Eufy Camera Corner Mount (Autodesk Fusion 360 design; units mm, degrees)
Autodesk Fusion 360 part; units mm, degrees
sketch "Sketch1" plane through (0, 0, 0) normal (0, 0, 1) x (1, 0, 0)
  line L0 (0, 0) -> (0, -37.5335) construction
  line L1 (31.3, -31.3) -> (31.3, 13.7)
  line L2 (31.3, -31.3) -> (2, -2)
  line L3 (-31.3, -31.3) -> (-31.3, 13.7)
  line L4 (-31.3, -31.3) -> (-2, -2)
  line L5 (31.3, 13.7) -> (-31.3, 13.7)
  arc A0 (2, -2) -> (-2, -2) centre (0, -2) ccw
  dimension "d1" = 62.6
  dimension "d2" = 45
  dimension "d4" = 90
  dimension "d5" = 2
  constraint coincident L0.start origin
  constraint vertical L0
  constraint vertical L1
  constraint symmetric L0 L1.start L3.start
  constraint symmetric L0 L1.end L3.end
  constraint coincident L0.start A0
  constraint midpoint L0.start A0
  constraint equal L2 L4
  constraint vertical L0.start A0.centre
  constraint horizontal L2.end A0.centre
  measures "d1" distance of L1.end L3.end
  measures "d2" distance of L1.start L1.end
  measures "d4" angle of L2 L4
  measures "d5" radius of A0
extrude "Extrude1" add sketch "Sketch1" along normal blind 56
sketch "Sketch2" plane through (0, 0, 0) normal (0.707107, -0.707107, 0) x (0.707107, 0.707107, 0)
  line L0 (-44.2649, 0) -> (-2.8284, 0)
  line L1 (-2.8284, 0) -> (-2.8284, 56)
  line L2 (-2.8284, 56) -> (-44.2649, 56)
  line L3 (-44.2649, 56) -> (-44.2649, 0)
  circle A0 centre (-25.8284, 41) radius 2
  circle A1 centre (-25.8284, 15) radius 2
  circle A2 centre (-25.8284, 15) radius 6.5
  circle A3 centre (-25.8284, 41) radius 6.5
  dimension "d8" = 15
  dimension "d10" = 4
  dimension "d11" = 15
  dimension "d12" = 23
  dimension "d15" = 13
  constraint equal A0 A1
  constraint vertical A0.centre A1.centre
  constraint concentric A1 A2
  constraint concentric A0 A3
  constraint equal A2 A3
  measures "d8" distance of L2 A0.centre
  measures "d10" diameter of A1
  measures "d11" distance of L0 A1.centre
  measures "d12" distance of L1 A0.centre
  measures "d15" diameter of A2
extrude "Extrude2" cut sketch "Sketch2" against normal blind 61.002 contours A0 | A1
extrude "Extrude3" cut sketch "Sketch2" along normal blind 17 from surface at -30 contours A2 | A3
sketch "Sketch3" plane through (0, 13.7, 0) normal (0, 1, 0) x (-1, 0, 0)
  line L0 (-31.3, 0) -> (31.3, 0)
  line L1 (31.3, 0) -> (31.3, 56)
  line L2 (31.3, 56) -> (-31.3, 56)
  line L3 (-31.3, 56) -> (-31.3, 0)
  line L4 (0, 56) -> (0, 42.8245) construction
  circle A0 centre (-22.5, 31) radius 1.5
  circle A1 centre (22.5, 31) radius 1.5
  circle A2 centre (0, 8.5) radius 1.5
  dimension "d19" = 25
  dimension "d20" = 45
  dimension "d21" = 3
  dimension "d30" = 8.5
  constraint midpoint L2 L4.start
  constraint perpendicular L2 L4
  constraint symmetric L4 A0 A1
  constraint equal A1 A2
  constraint vertical origin A2.centre
  measures "d19" distance of L2 A0.centre
  measures "d20" distance of A0.centre A1.centre
  measures "d21" diameter of A0
  measures "d30" distance of L0 A2.centre
hole "Hole1" at (22.5, 13.7, 31) at (-22.5, 13.7, 31) at (0, 13.7, 8.5) direction (0, -1, 0) diameter 2.529 depth 25 tip angle 118
thread "Thread1" "ISO Metric profile 3.0 M3x0.5 M3x0.5 6H" thread offset 0 thread depth 7.4
fillet "Fillet1" radius 9 4 edges at (31.3, -8.8, 56) (-31.3, -8.8, 56) (-31.3, -8.8, 0) (31.3, -8.8, 0)
mirror "Mirror1" about plane through (0, 0, 0) normal (1, 0, 0) of "Extrude2", "Extrude3"
equation "d11 = d8"
named bodies: "Eufy Camera Corner Mount"
